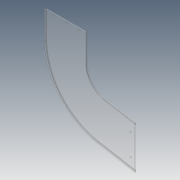
# Autodesk Inventor part: GE-12071-01
Saved by Autodesk Inventor 2012 (Build 160160000, 160)
## iProperties
Created: 2011-09-22
Part Number: GE-12071-01
Document SubType Name: Modeling
Designer: dfoster
Density: 1 g/cm^3
Description: Chute 1, Side
Material: Default
Title: Chute 1, Side
Author: dfoster
Autodesk Inventor part; units mm, degrees
ref_plane "YZ Plane" through (0, 0, 0) normal (1, 0, 0) x (0, 1, 0)
ref_plane "XZ Plane" through (0, 0, 0) normal (0, 1, 0) x (-1, 0, 0)
ref_plane "XY Plane" through (0, 0, 0) normal (0, 0, 1) x (1, 0, 0)
sketch "Sketch1" plane through (0, 0, 0) normal (0, 0, 1) x (1, 0, 0)
  line L0 (0, 0) -> (0, -161.1088)
  line L1 (0, 0) -> (244.475, 0)
  line L2 (244.475, 0) -> (244.475, -161.1088)
  line L3 (349.4217, -286.1793) -> (527.05, -317.5)
  line L4 (527.05, -317.5) -> (527.05, -565.7464)
  line L5 (527.05, -565.7464) -> (306.969, -526.9402)
  arc A0 (244.475, -161.1088) -> (349.4217, -286.1793) centre (371.475, -161.1088) ccw
  arc A1 (0, -161.1088) -> (306.969, -526.9402) centre (371.475, -161.1088) ccw
  dimension "d0" = 244.475
  dimension "d1" = 244.475
  dimension "d2" = 100
  dimension "d3" = 127
  dimension "d4" = 371.475
  dimension "d5" = 317.5
  dimension "d6" = 527.05
  constraints: 12 end point, 4 point on circle, 4 tangent, 2 centre point, 2 parallel, 2 perpendicular, 1 vertical
  measures "d0" distance of L0.start L1.end
  measures "d1" distance between parallel lines of L5 L3
  measures "d2" angle of L5 L0
  measures "d3" radius of A0
  measures "d4" radius of A1
  measures "d5" distance from line of L3.end L1
  measures "d6" distance between parallel lines of L4 L0
extrude "Extrusion1" add sketch "Sketch1" along normal blind 6.35
sketch "Sketch3" plane through (0, 0, 0) normal (0, 0, -1) x (-1, 0, 0)
  line L0 (0, 0) -> (0, -161.1088) projected
  line L1 (-244.475, 0) -> (0, 0) projected
  line L2 (-244.475, -161.1088) -> (-244.475, 0) projected
  arc A0 (-349.4217, -286.1793) -> (-244.475, -161.1088) centre (-371.475, -161.1088) ccw projected
  line L3 (-527.05, -317.5) -> (-349.4217, -286.1793) projected
  line L4 (-527.05, -565.7464) -> (-527.05, -317.5) projected
  line L5 (-306.969, -526.9402) -> (-527.05, -565.7464) projected
  arc A1 (-306.969, -526.9402) -> (0, -161.1088) centre (-371.475, -161.1088) ccw projected
  line L6 (-4.7625, 0) -> (-4.7625, -161.1088)
  arc A2 (-307.796, -522.2501) -> (-4.7625, -161.1088) centre (-371.475, -161.1088) ccw
  line L7 (-307.796, -522.2501) -> (-527.05, -560.9105)
  line L8 (-527.05, -322.336) -> (-348.5947, -290.8695)
  arc A3 (-348.5947, -290.8695) -> (-239.7125, -161.1088) centre (-371.475, -161.1088) ccw
  line L9 (-239.7125, -161.1088) -> (-239.7125, 0)
  line L10 (-236.5375, 0) -> (-236.5375, -161.1088)
  arc A4 (-348.0433, -293.9962) -> (-236.5375, -161.1088) centre (-371.475, -161.1088) ccw
  line L11 (-348.0433, -293.9962) -> (-527.05, -325.5599)
  line L12 (-7.9375, 0) -> (-7.9375, -161.1088)
  arc A5 (-308.3474, -519.1233) -> (-7.9375, -161.1088) centre (-371.475, -161.1088) ccw
  line L13 (-308.3474, -519.1233) -> (-527.05, -557.6865)
  line L14 (-239.7125, 0) -> (-236.5375, 0)
  line L15 (-4.7625, 0) -> (-7.9375, 0)
  line L16 (-527.05, -322.336) -> (-527.05, -325.5599)
  line L17 (-527.05, -560.9105) -> (-527.05, -557.6865)
  dimension "d21" = 4.7625
  dimension "d23" = 4.7625
  dimension "d24" = 4.7625
  dimension "d25" = 4.7625
  dimension "d26" = 4.7625
  dimension "d27" = 4.7625
  dimension "d28" = 3.175
  dimension "d29" = 3.175
  dimension "d30" = 3.175
  dimension "d31" = 3.175
  constraints: 24 end point, 8 point on circle, 5 point on line, 4 centre point, 3 perpendicular, 2 parallel, 1 vertical, 2 other
  measures "d21" distance between parallel lines of L2 L9
  measures "d23" distance between parallel lines of L3 L8
  measures "d24" distance between parallel lines of L6 L0
  measures "d25" radial gap between concentric circles of A2 A1
  measures "d26" distance between parallel lines of L7 L5
  measures "d27" radial gap between concentric circles of A0 A3
  measures "d28" distance between parallel lines of L9 L10
  measures "d29" distance between parallel lines of L12 L6
  measures "d30" distance between parallel lines of L11 L8
  measures "d31" distance between parallel lines of L7 L13
extrude "Extrusion3" cut sketch "Sketch3" against normal blind 3.175 contours L6 A2 L7 L4 L13 A5 L12 L1 | L10 A4 L11 L4 L8 A3 L9 L1
hole "Hole1" at (498.475, -377.825, 6.35) direction (0, 0, -1) diameter 6.731 depth 25.4 tip angle 118
pattern_linear "Rectangular Pattern1" count 2 spacing 127 along (0, -1, 0) of "Hole1"
hole "Hole2" at (200.025, -12.7, 6.35) direction (0, 0, -1) diameter 6.731 depth 25.4 tip angle 118
pattern_linear "Rectangular Pattern2" count 3 spacing 76.2 along (-1, 0, 0) of "Hole2"
equation "\"d1\" = d0"
equation "\"d4\" = d3 + d0"
equation "\"d23\" = d21"
equation "\"d24\" = d21"
equation "\"d25\" = d21"
equation "\"d26\" = d21"
equation "\"d27\" = d21"
body "Solid1"
